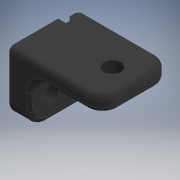
# Autodesk Inventor part: Threaded Rod Guide
Saved by Autodesk Inventor 2020.2 (Build 242310000, 310)
## iProperties
Created: 2019-11-16
Part Number: Threaded Rod Guide
Material: ABS Plastic
Document SubType Name: Modeling
Designer: Richard Hall
Density: 1.06 g/cm^3
Appearance: Rubber - Black
Author: Richard Hall
Autodesk Inventor part; units mm, degrees
ref_plane "YZ Plane" through (0, 0, 0) normal (1, 0, 0) x (0, 1, 0)
ref_plane "XZ Plane" through (0, 0, 0) normal (0, 1, 0) x (-1, 0, 0)
ref_plane "XY Plane" through (0, 0, 0) normal (0, 0, 1) x (1, 0, 0)
sketch "Sketch1" plane through (0, 0, 0) normal (0, 1, 0) x (-1, 0, 0)
  line L0 (15, 11) -> (2.2, 11)
  line L1 (-15, 11) -> (-15, -5.2)
  line L2 (-15, -11) -> (-9.2, -11)
  line L3 (15, -11) -> (15, 11)
  line L4 (15, 11) -> (-15, -11) construction
  line L5 (-15, 11) -> (15, -11) construction
  circle A0 centre (-7.2, 0) radius 2.75
  line L6 (-9.2, -11) -> (15, -11)
  line L7 (-15, -5.2) -> (-15, -11)
  line L8 (2.2, 11) -> (-15, 11)
  point P0 (0, 0)
  point P1 (0, 0)
  dimension "d0" = 30
  dimension "d1" = 22
  dimension "d2" = 5.5
  dimension "d4" = 22.2
  constraints: 18 end point, 6 parallel, 4 perpendicular, 3 midpoint, 2 horizontal, 1 centre point, 1 horizontal alignment
  measures "d0" distance of L3.start L2.start
  measures "d1" distance of L2.start L1.start
  measures "d2" diameter of A0
  measures "d4" distance from line of L3 A0.centre
extrude "Extrusion1" add sketch "Sketch1" against normal mid plane 20
ref_plane "Work Plane1" through (-8, -10, -11) normal (-1, 0, 0) x (0, 0, 1)
sketch "Sketch2" plane through (-8, -10, -11) normal (-1, 0, 0) x (0, 0, 1)
  line L0 (8.7074, 0) -> (22, 0)
  line L1 (0, 0) -> (0, 20) projected
  line L2 (17.8289, 0) -> (0, 0)
  line L3 (0, 0) -> (0, 15)
  line L4 (0, 15) -> (22, 15)
  line L5 (22, 15) -> (22, 0)
  line L6 (22, 0) -> (22, 20) projected
  line L7 (22, 0) -> (22, 20) projected
  line L8 (22, 0) -> (0, 0) projected
  point P0 (11, 10)
  dimension "d28" = 5
  constraints: 10 end point, 3 collinear, 2 parallel, 1 horizontal, 1 perpendicular, 1 point on line
  measures "d28" distance from line of L1.end L4
extrude "Extrusion2" cut sketch "Sketch2" against normal blind 33.75
fillet "Fillet1" radius 5 1 edges at (-8, 5, 0)
sketch "Sketch3" plane through (-8, -10, -11) normal (1, 0, 0) x (0, 0, -1)
  line L0 (0, 0) -> (-22, 0) projected
  point P0 (-11, 10)
  point P1 (-16, 7)
  dimension "d29" = 5
  dimension "d30" = 7
  measures "d29" horizontal distance of point (-11, 10) point (-16, 7)
  measures "d30" distance from line of L0 point (-16, 7)
hole "Hole1" at (-8, -3, 5) direction (-1, 0, 0) diameter 5.5 end through all start extended yes counterbore diameter 11 counterbore depth 0.001 clearance for "Socket Head Cap Screw" size "M5" standard "Ansi Metric M Profile"
fillet "Fillet2" radius 5 4 edges at (-11.5, -10, 11) (-11.5, -10, -11) (15, 7.5, -11) (15, 7.5, 11)
fillet "Fillet3" radius 1.5 7 edges at (-8, -10, 0) (-8, -8.5355, 9.5355) (-8, -2.5, 11) (-6.5355, 3.5355, 11) (3.5, 5, 11) (-2.5, 10, 11) (-2.5, 10, -11)
sketch "Sketch5" plane through (0, 10, 0) normal (0, 1, 0) x (1, 0, 0)
  line L0 (-15, 4.75) -> (-11.25, 4.75)
  line L1 (-11.25, 4.75) -> (-15, 8.5)
  line L2 (-15, 9.5) -> (-15, -9.5) construction
  line L3 (-15, -7.75) -> (-15, -2.25) projected
  line L4 (-15, 8.5) -> (-15, 4.75)
  line L5 (-12.5, 4.75) -> (-12.5, 6)
  point P0 (0, 0)
  point P1 (-15, -5)
  dimension "d31" = 9.75
  dimension "d33" = 45
  dimension "d34" = 3.75
  dimension "d37" = 2.5
  constraints: 8 end point, 4 point on line, 1 horizontal, 1 midpoint, 1 vertical
  measures "d31" distance from line of L0 point (-15, -5)
  measures "d33" angle of L0 L1
  measures "d34" distance from line of L1.end L0
  measures "d37" distance between parallel lines of L2 L5
extrude "Extrusion4" cut sketch "Sketch5" against normal through all contours L4 L1 L5 L0
fillet "Fillet4" radius 2 4 edges at (-15, 10, -9) (-15, 1.75, -11) (-15, -7.5, -10.3301) (-15, 9.5607, -10.5607)
body "Solid1"
